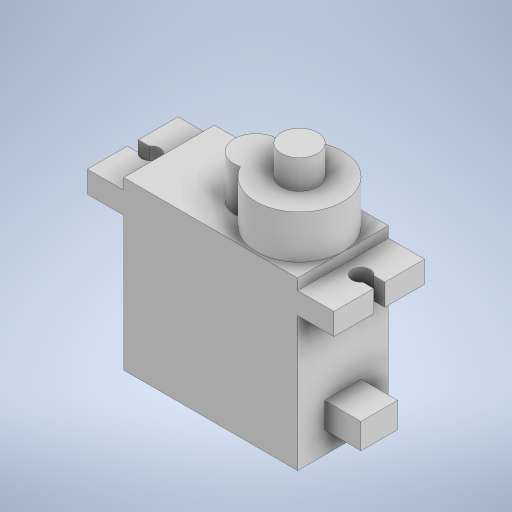
# Autodesk Inventor part: S
Saved by Autodesk Inventor 2023 (Build 270158000, 158)
## iProperties
Created: 2022-04-07
Part Number: S
Material: Generic
Document SubType Name: Modeling
Designer: kao91
Density: 1 g/cm^3
Appearance: Default
Author: kao91
Autodesk Inventor part; units mm, degrees
ref_plane "YZ Plane" through (0, 0, 0) normal (1, 0, 0) x (0, 1, 0)
ref_plane "XZ Plane" through (0, 0, 0) normal (0, 1, 0) x (-1, 0, 0)
ref_plane "XY Plane" through (0, 0, 0) normal (0, 0, 1) x (1, 0, 0)
sketch "Sketch1" plane through (0, 0, 0) normal (0, 0, 1) x (1, 0, 0)
  line L0 (-2.5, 0) -> (2.5, 0)
  line L1 (2.5, 0) -> (2.5, -4)
  line L2 (2.5, -4) -> (-2.5, -4)
  line L3 (-2.5, -4) -> (-2.5, 0)
  line L4 (6, -4) -> (-9, -4)
  line L5 (-9, -4) -> (-9, -10)
  line L6 (-9, -10) -> (6, -10)
  line L7 (6, -10) -> (6, -4)
  line L8 (6, -10) -> (-18, -10)
  line L9 (-18, -10) -> (-18, -33)
  line L10 (-18, -33) -> (6, -33)
  line L11 (6, -33) -> (6, -10)
  line L12 (-18, -11.5) -> (-23, -11.5)
  line L13 (-23, -11.5) -> (-23, -14.5)
  line L14 (-23, -14.5) -> (-18, -14.5)
  line L15 (-18, -14.5) -> (-18, -11.5)
  line L16 (6, -11.5) -> (11, -11.5)
  line L17 (11, -11.5) -> (11, -14.5)
  line L18 (11, -14.5) -> (6, -14.5)
  line L19 (6, -14.5) -> (6, -11.5)
  line L20 (-6, -33) -> (-6, -10) construction
  point P0 (0, 0)
  point P1 (0, -4)
  point P2 (11, -13)
  point P3 (-23, -13)
  point P4 (-9, -7)
  point P5 (0, 0)
  point P6 (-18, -14.5)
  point P7 (6, -14.5)
  dimension "d0" = 5
  dimension "d1" = 4
  dimension "d2" = 6
  dimension "d3" = 6
  dimension "d4" = 24
  dimension "d6" = 34
  dimension "d7" = 9
  dimension "d8" = 1.5
  dimension "d9" = 3
  dimension "d31" = 18.5
  constraints: 42 end point, 10 parallel, 7 midpoint, 5 horizontal, 5 perpendicular, 4 point on line, 1 coincident, 1 collinear, 1 other
  measures "d0" distance of L1.end L2.end
  measures "d1" distance of L0.end L1.end
  measures "d2" distance of L5.end L4.end
  measures "d3" distance from line of L7 point (0, -4)
  measures "d4" distance of L9.end L10.end
  measures "d6" distance of point (11, -13) point (-23, -13)
  measures "d7" horizontal distance of L8.end point (-9, -7)
  measures "d8" distance from line of L16 L6.end
  measures "d9" distance of L16.end L17.end
  measures "d31" distance between parallel lines of L10 L18
extrude "Extrusion1" add sketch "Sketch1" along normal mid plane 12.5 contours L6 L11 L10 L9 L8 | L16 L17 L18 L11 | L9 L14 L13 L12
sketch "Sketch2" plane through (-18, -10, 6.25) normal (0, 1, 0) x (1, 0, 0)
  circle A0 centre (18, 6.25) radius 6
  line L0 (24, 12.5) -> (24, 0) construction
  circle A1 centre (12, 6.25) radius 3
  line L1 (0, 12.5) -> (0, 0) construction
  point P0 (9, 6.25)
  point P1 (0, 6.25)
  point P2 (12.75, 9.1547)
  point P3 (12.75, 3.3453)
  dimension "d12" = 9
  constraints: 1 coincident, 1 midpoint, 1 vertical, 6 other
  measures "d12" distance of point (9, 6.25) point (0, 6.25)
extrude "Extrusion2" add sketch "Sketch2" along normal blind 6
sketch "Sketch3" plane through (-18, -4, 6.25) normal (0, 1, 0) x (1, 0, 0)
  circle A0 centre (18, 6.25) radius 2.5
  dimension "d15" = 5
  constraints: 1 centre point, 1 coincident
  measures "d15" diameter of A0
extrude "Extrusion3" add sketch "Sketch3" along normal blind 4
sketch "Sketch4" plane through (6, -33, 6.25) normal (1, 0, 0) x (0, 0, -1)
  line L0 (3.7222, 6.5) -> (8.7778, 6.5)
  line L1 (8.7778, 6.5) -> (8.7778, 3)
  line L2 (8.7778, 3) -> (3.7222, 3)
  line L3 (3.7222, 3) -> (3.7222, 6.5)
  line L4 (0, 0) -> (0, 18.5) construction
  line L5 (0, 6.5) -> (3.7222, 6.5) construction
  line L6 (8.7778, 6.5) -> (12.5, 6.5) construction
  line L7 (12.5, 18.5) -> (12.5, 0) construction
  line L8 (12.5, 0) -> (0, 0) construction
  line L9 (12.5, 18.5) -> (0, 18.5) construction
  point P0 (6.25, 33)
  point P1 (6.25, 18.5)
  point P2 (6.25, 6.5)
  dimension "d18" = 3
  dimension "d19" = 12
  constraints: 12 end point, 3 point on line, 2 midpoint, 2 parallel, 2 perpendicular, 1 collinear, 1 horizontal
  measures "d18" distance between parallel lines of L8 L2
  measures "d19" distance of point (6.25, 18.5) point (6.25, 6.5)
extrude "Extrusion4" add sketch "Sketch4" along normal blind 5
sketch "Sketch5" plane through (6, -11.5, 6.25) normal (0, 1, 0) x (1, 0, 0)
  line L0 (-29, 12.5) -> (-29, 0) construction
  line L1 (-24, 0) -> (-29, 0) construction
  line L2 (-24, 12.5) -> (-24, 0) construction
  line L3 (-29, 12.5) -> (-24, 12.5) construction
  line L4 (0, 12.5) -> (0, 0) construction
  line L5 (5, 0) -> (0, 0) construction
  line L6 (5, 12.5) -> (5, 0) construction
  line L7 (0, 12.5) -> (5, 12.5) construction
  line L8 (-29, 6.25) -> (5, 6.25) construction
  line L9 (5, 3.7222) -> (5, 8.7778) construction
  circle A0 centre (-26.5, 6.25) radius 1.25
  circle A1 centre (2.5, 6.25) radius 1.25
  line L10 (-12, 6.25) -> (-12, 12.5) construction
  line L11 (-27.5, 5.5) -> (-29, 5.5)
  line L12 (-29, 5.5) -> (-29, 7)
  line L13 (-29, 7) -> (-27.5, 7)
  line L14 (-27.5, 7) -> (-27.5, 5.5)
  line L15 (3.5, 7) -> (5, 7)
  line L16 (5, 7) -> (5, 5.5)
  line L17 (5, 5.5) -> (3.5, 5.5)
  line L18 (3.5, 5.5) -> (3.5, 7)
  line L19 (3.5, 7) -> (5, 5.5) construction
  line L20 (5, 7) -> (3.5, 5.5) construction
  point P0 (-6, 6.25)
  point P1 (4.25, 6.25)
  point P2 (3.5, 5.5)
  dimension "d22" = 2.5
  dimension "d23" = 29
  dimension "d24" = 1.5
  dimension "d25" = 1.5
  constraints: 24 end point, 5 midpoint, 5 point on line, 4 parallel, 2 horizontal, 2 perpendicular, 1 symmetric about line, 1 vertical, 7 other
  measures "d23" distance of point (2.5, 6.25) point (-26.5, 6.25)
  measures "d24" distance of L13.end L11.start
  measures "d25" distance of L17.end L15.start
extrude "Extrusion5" cut sketch "Sketch5" against normal blind 3
sketch "Sketch6" plane through (0, 0, 0) normal (0, 1, 0) x (1, 0, 0)
  circle A0 centre (0, 0) radius 2.5 projected
  circle A1 centre (0, 0) radius 10
  point P0 (0, 0)
  dimension "d28" = 20
  constraints: 1 centre point, 1 coincident
  measures "d28" diameter of A1
body "Solid1"
